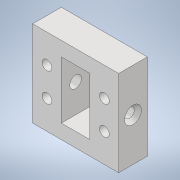
# Autodesk Inventor part: Tensor
Saved by Autodesk Inventor 2022.3 (Build 263350000, 350)
## iProperties
Created: 2023-05-20
Part Number: Tensor
Material: Generic
Document SubType Name: Modeling
Designer: Manuel Hueso Béjar
Density: 1 g/cm^3
Appearance: Default
Author: Manuel Hueso Béjar
Autodesk Inventor part; units mm, degrees
ref_plane "YZ Plane" through (0, 0, 0) normal (1, 0, 0) x (0, 1, 0)
ref_plane "XZ Plane" through (0, 0, 0) normal (0, 1, 0) x (-1, 0, 0)
ref_plane "XY Plane" through (0, 0, 0) normal (0, 0, 1) x (1, 0, 0)
sketch "Sketch1" plane through (0, 0, 0) normal (0, 1, 0) x (-1, 0, 0)
  line L0 (-15, 5) -> (15, 5)
  line L1 (15, 5) -> (15, -5)
  line L2 (15, -5) -> (-15, -5)
  line L3 (-15, -5) -> (-15, 5)
  line L4 (-15, 5) -> (15, -5) construction
  line L5 (15, 5) -> (-15, -5) construction
  point P0 (0, 0)
  dimension "d0" = 30
  dimension "d1" = 10
  constraints: 12 end point, 2 midpoint, 2 parallel, 1 horizontal, 1 perpendicular
  measures "d0" distance of L1.end L2.end
  measures "d1" distance of L0.end L1.end
extrude "Extrusion1" add sketch "Sketch1" along normal blind 30
sketch "Sketch2" plane through (15, 0, -5) normal (0, 0, -1) x (-1, 0, 0)
  line L0 (0, 0) -> (0, 30) projected
  line L1 (0, 30) -> (30, 30) projected
  line L2 (0, 0) -> (30, 30)
  line L3 (10, 5) -> (20, 5)
  line L4 (20, 5) -> (20, 25)
  line L5 (20, 25) -> (10, 25)
  line L6 (10, 25) -> (10, 5)
  line L7 (10, 5) -> (20, 25) construction
  line L8 (20, 5) -> (10, 25) construction
  point P0 (15, 0)
  point P1 (15, 15)
  dimension "d4" = 10
  dimension "d5" = 20
  constraints: 14 end point, 3 midpoint, 2 parallel, 1 horizontal, 1 perpendicular
  measures "d4" distance of L5.end L4.end
  measures "d5" distance of L4.end L3.end
extrude "Extrusion2" cut sketch "Sketch2" against normal through all contours L6 L5 L4 L2 | L2 L4 L3 L6
sketch "Sketch3" plane through (15, 0, 5) normal (1, 0, 0) x (0, 0, -1)
  line L0 (10, 0) -> (0, 0) projected
  line L1 (0, 30) -> (10, 30) projected
  line L2 (0, 0) -> (10, 30)
  line L3 (5, 15) -> (17.6725, 15)
  point P0 (5, 0)
  constraints: 4 end point, 1 horizontal, 1 midpoint
hole "Hole1" at (15, 15, 0) direction (-1, 0, 0) diameter 3.4 depth 10 countersink diameter 5.9 countersink angle 90
sketch "Sketch4" plane through (-5, 5, -5) normal (1, 0, 0) x (0, 0, -1)
  line L0 (-10, 0) -> (-10, 20) projected
  line L1 (0, 20) -> (-10, 20) projected
  line L2 (-10, 0) -> (0, 20)
  line L3 (-5, 10) -> (5, 10)
  point P0 (-5, -5)
  dimension "d15" = 10
  constraints: 4 end point, 1 horizontal, 1 midpoint
  measures "d15" distance of L3.start L3.end
hole "Hole2" at (-5, 15, 0) direction (-1, 0, 0) diameter 3.4 depth 9 counterbore diameter 4.1 counterbore depth 5.1
sketch "Sketch5" plane through (15, 0, -5) normal (0, 0, -1) x (-1, 0, 0)
  line L0 (30, 0) -> (0, 0) projected
  line L1 (30, 0) -> (30, 30) projected
  line L2 (0, 0) -> (30, 30)
  line L3 (5, 10) -> (25, 10)
  line L4 (25, 10) -> (25, 20)
  line L5 (25, 20) -> (5, 20)
  line L6 (5, 20) -> (5, 10)
  line L7 (5, 10) -> (25, 20) construction
  line L8 (25, 10) -> (5, 20) construction
  point P0 (15, 0)
  point P1 (15, 15)
  dimension "d23" = 20
  dimension "d24" = 10
  constraints: 14 end point, 3 midpoint, 2 parallel, 1 horizontal, 1 perpendicular
  measures "d23" distance of L5.end L4.end
  measures "d24" distance of L4.end L3.end
hole "Hole3" at (10, 20, -5) at (10, 10, -5) at (-10, 10, -5) at (-10, 20, -5) direction (0, 0, 1) diameter 3.4 end through all countersink diameter 5.9 countersink angle 90
fillet "Fillet1" radius 6 6 edges at (15, 30, 0) (-15, 30, 0) (15, 0, 0) (-15, 0, 0) (0, 30, -5) (0, 0, -5)
fillet "Fillet2" radius 2 6 edges at (13.2426, 28.2426, -3.2426) (13.2426, 1.7574, -3.2426) (15, 15, -5) (-13.2426, 28.2426, -3.2426) (-13.2426, 1.7574, -3.2426) (-15, 15, -5)
body "Solid1"
